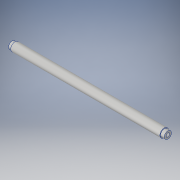
# Autodesk Inventor part: Idle Drive Axle
Saved by Autodesk Inventor 2019.4 (Build 234330000, 330)
## iProperties
Created: 2020-01-24
Part Number: Idle Drive Axle
Material: Aluminum 6061
Document SubType Name: Modeling
Designer: admin
Density: 2.7 g/cm^3
Appearance: Aluminum - Flat
Author: admin
Autodesk Inventor part; units mm, degrees
ref_plane "YZ Plane" through (0, 0, 0) normal (1, 0, 0) x (0, 1, 0)
ref_plane "XZ Plane" through (0, 0, 0) normal (0, 1, 0) x (-1, 0, 0)
ref_plane "XY Plane" through (0, 0, 0) normal (0, 0, 1) x (1, 0, 0)
sketch "Sketch1" plane through (0, 0, 0) normal (0, 0, 1) x (1, 0, 0)
  line L0 (0, 0) -> (0, 5)
  line L1 (0, 5) -> (4, 5)
  line L2 (4, 5) -> (4, 6)
  line L3 (4, 6) -> (210.2, 6)
  line L4 (210.2, 6) -> (210.2, 5)
  line L5 (210.2, 5) -> (215.2, 5)
  line L6 (215.2, 5) -> (215.2, 0)
  line L7 (215.2, 0) -> (0, 0)
  dimension "d0" = 4
  dimension "d1" = 206.2
  dimension "d2" = 5
  dimension "d3" = 5
  dimension "d4" = 6
  dimension "d5" = 5
  constraints: 16 end point, 7 perpendicular, 1 vertical
  measures "d0" distance of L0.end L1.end
  measures "d1" distance between parallel lines of L4 L2
  measures "d2" distance of L4.end L5.end
  measures "d3" distance between parallel lines of L7 L1
  measures "d4" distance between parallel lines of L7 L3
  measures "d5" distance between parallel lines of L7 L5
revolve "Revolution1" add sketch "Sketch1" angle 360 about axis through (215.2, 0, 0) along (-1, 0, 0)
sketch "Sketch2" plane through (215.2, 0, 0) normal (1, 0, 0) x (0, 0, -1)
  circle A0 centre (0, 0) radius 5 projected
  constraints: 1 coincident
hole "Hole1" at (215.2, 0, 0) direction (-1, 0, 0) diameter 5 end through all
body "Solid1"
